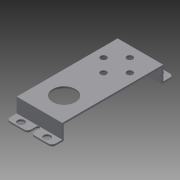
# Autodesk Inventor part: Quarter-Scale Servo Front Mount Bracket
Saved by Autodesk Inventor 2014 SP2 (Build 180246200, 246)
## iProperties
Created: 2014-09-14
Part Number: Quarter-Scale Servo Front Mount Bracket
Material: Generic
Document SubType Name: Modeling
Designer: Allison
Density: 1 g/cm^3
Appearance: Default
Author: Allison
Autodesk Inventor part; units mm, degrees
ref_plane "YZ Plane" through (0, 0, 0) normal (1, 0, 0) x (0, 1, 0)
ref_plane "XZ Plane" through (0, 0, 0) normal (0, 1, 0) x (-1, 0, 0)
ref_plane "XY Plane" through (0, 0, 0) normal (0, 0, 1) x (1, 0, 0)
sketch "Sketch1" plane through (0, 0, 0) normal (0, 1, 0) x (-1, 0, 0)
  line L0 (0.3746, 1.6788) -> (0.3747, -4.4196)
  line L1 (3.5497, -7.5946) -> (5.0483, -7.5946)
  arc A0 (7.6772, -6.364) -> (5.0483, -6.4323) centre (6.3183, -4.6863) ccw
  line L2 (7.6772, -7.5946) -> (20.7963, -7.5946)
  arc A1 (23.4251, -6.4323) -> (20.7962, -6.364) centre (22.1552, -4.6863) ccw
  line L3 (23.4252, -7.5946) -> (24.9238, -7.5946)
  line L4 (20.7963, 66.2432) -> (7.6772, 66.2432)
  arc A2 (5.0483, 65.0809) -> (7.6772, 65.0126) centre (6.3183, 63.3349) ccw
  line L5 (5.0483, 66.2432) -> (3.5496, 66.2432)
  line L6 (24.9237, 66.2432) -> (23.4252, 66.2432)
  arc A3 (20.7962, 65.0126) -> (23.4251, 65.0809) centre (22.1552, 63.3349) ccw
  circle A4 centre (14.2367, 45.0719) radius 6.9278
  arc A5 (1.9876, 15.9067) -> (5.1626, 12.7318) centre (5.1626, 15.9067) ccw
  line L7 (5.1626, 12.7318) -> (23.3109, 12.7318)
  arc A6 (23.3109, 12.7318) -> (26.4859, 15.9068) centre (23.3109, 15.9068) ccw
  line L8 (26.4859, 15.9068) -> (26.4859, 45.1707)
  arc A7 (26.4859, 45.1707) -> (1.9876, 45.1707) centre (14.2367, 45.0719) ccw
  line L9 (1.9876, 45.1707) -> (1.9876, 15.9067)
  arc A8 (27.813, 45.1759) -> (0.6604, 45.1759) centre (14.2367, 45.0719) ccw
  circle A9 centre (14.2367, 45.0719) radius 6.9278
  line L10 (0.3746, 66.2432) -> (13.2207, 66.2432)
  line L11 (13.2207, 66.2432) -> (13.2207, 60.019)
  line L12 (13.2207, 60.019) -> (0.3746, 60.019)
  line L13 (0.3746, 60.019) -> (0.3746, 66.2432)
  line L14 (0.3746, 60.019) -> (13.2207, 60.019)
  line L15 (13.2207, 60.019) -> (13.2207, 59.1663)
  line L16 (13.2207, 59.1663) -> (0.3746, 59.1663)
  line L17 (0.3746, 59.1663) -> (0.3746, 60.019)
  line L18 (14.2367, 45.0719) -> (14.2367, 66.2432)
  line L19 (28.0988, 66.2432) -> (15.2527, 66.2432)
  line L20 (15.2527, 66.2432) -> (15.2527, 60.019)
  line L21 (28.0988, 60.019) -> (28.0988, 66.2432)
  line L22 (28.0988, 60.019) -> (15.2527, 60.019)
  line L23 (15.2527, 60.019) -> (15.2527, 59.1663)
  line L24 (15.2527, 59.1663) -> (28.0988, 59.1663)
  line L25 (28.0988, 59.1663) -> (28.0988, 60.019)
  circle A10 centre (6.3183, 63.3349) radius 2.159
  circle A11 centre (22.1552, 63.3349) radius 2.159
  line L26 (0.3746, 66.2432) -> (0.3746, -7.5946)
  line L27 (0.3746, 29.3243) -> (28.0988, 29.3243)
  line L28 (20.7963, -7.5946) -> (7.6772, -7.5946)
  arc A12 (7.6772, -6.364) -> (5.0483, -6.4323) centre (6.3182, -4.6863) ccw
  line L29 (5.0483, -7.5946) -> (3.5497, -7.5946)
  line L30 (24.9238, -7.5946) -> (23.4252, -7.5946)
  arc A13 (23.4251, -6.4323) -> (20.7962, -6.364) centre (22.1551, -4.6863) ccw
  line L31 (0.3746, -7.5946) -> (13.2207, -7.5946)
  line L32 (13.2207, -7.5946) -> (13.2207, -1.3704)
  line L33 (13.2207, -1.3704) -> (0.3746, -1.3704)
  line L34 (0.3746, -1.3704) -> (0.3746, -7.5946)
  line L35 (0.3746, -1.3704) -> (13.2207, -1.3704)
  line L36 (13.2207, -1.3704) -> (13.2207, -0.5177)
  line L37 (13.2207, -0.5177) -> (0.3746, -0.5177)
  line L38 (0.3746, -0.5177) -> (0.3746, -1.3704)
  line L39 (28.0988, -1.3704) -> (28.0988, -7.5946)
  line L40 (28.0988, -7.5946) -> (15.2527, -7.5946)
  line L41 (15.2527, -7.5946) -> (15.2527, -1.3704)
  line L42 (28.0988, -1.3704) -> (15.2527, -1.3704)
  line L43 (15.2527, -0.5177) -> (28.0988, -0.5177)
  line L44 (15.2527, -1.3704) -> (15.2527, -0.5177)
  line L45 (28.0988, -0.5177) -> (28.0988, -1.3704)
  circle A14 centre (6.3182, -4.6863) radius 2.159
  circle A15 centre (22.1551, -4.6863) radius 2.159
  line L46 (28.0988, -7.5946) -> (15.2527, -7.5946)
  line L47 (15.2527, -7.5946) -> (15.2527, -1.3704)
  line L48 (15.2527, -1.3704) -> (28.0988, -1.3704)
  line L49 (28.0988, -1.3704) -> (28.0988, -7.5946)
  line L50 (13.2207, -7.5946) -> (0.3746, -7.5946)
  line L51 (0.3746, -7.5946) -> (0.3746, -1.3704)
  line L52 (0.3746, -1.3704) -> (13.2207, -1.3704)
  line L53 (13.2207, -1.3704) -> (13.2207, -7.5946)
  line L54 (28.0988, 66.2432) -> (15.2527, 66.2432)
  line L55 (15.2527, 66.2432) -> (15.2527, 60.019)
  line L56 (15.2527, 60.019) -> (28.0988, 60.019)
  line L57 (28.0988, 60.019) -> (28.0988, 66.2432)
  point P0 (0, 0)
  point P1 (0, 20.6785)
  point P2 (14.2367, -7.5946)
  constraints: 116 end point, 25 symmetric about line, 20 point on circle, 16 centre point, 11 parallel, 6 perpendicular, 5 horizontal, 4 coincident, 2 midpoint, 1 concentric, 4 other
extrude "Extrusion1" add sketch "Sketch1" along normal blind 1 contours L41 L42 L39 L40 L3 L2 | L4 L19 L6 L21 L22 L20 | L33 L32 L2 L31 L1 L26 L0 | L13 L10 L5 L4 L11 L12
sketch "Sketch2" plane through (0, 0, 0) normal (0, -1, 0) x (1, 0, 0)
  circle A0 centre (-22.1552, 63.3349) radius 2.159 projected
  line L0 (-28.0988, 66.2432) -> (-15.2527, 66.2432) projected
  line L1 (-28.0988, 60.019) -> (-28.0988, 66.2432) projected
  line L2 (-15.2527, 60.019) -> (-28.0988, 60.019) projected
  line L3 (-15.2527, 66.2432) -> (-15.2527, 60.019) projected
  circle A1 centre (-6.3183, 63.3349) radius 2.159 projected
  line L4 (-0.3746, 66.2432) -> (-0.3746, 60.019) projected
  line L5 (-13.2207, 66.2432) -> (-0.3746, 66.2432) projected
  line L6 (-13.2207, 60.019) -> (-13.2207, 66.2432) projected
  line L7 (-0.3746, 60.019) -> (-13.2207, 60.019) projected
  circle A2 centre (-22.1551, -4.6863) radius 2.159 projected
  line L8 (-15.2527, -1.3704) -> (-15.2527, -7.5946) projected
  line L9 (-28.0988, -1.3704) -> (-15.2527, -1.3704) projected
  line L10 (-28.0988, -7.5946) -> (-28.0988, -1.3704) projected
  line L11 (-15.2527, -7.5946) -> (-28.0988, -7.5946) projected
  line L12 (-28.0988, 60.019) -> (-0.3746, 60.019)
  line L13 (-0.3746, 60.019) -> (-0.3746, 59.13)
  line L14 (-0.3746, 59.13) -> (-28.0988, 59.13)
  line L15 (-28.0988, 59.13) -> (-28.0988, 60.019)
  line L16 (-28.0988, -1.3704) -> (-0.3746, -1.3704)
  line L17 (-0.3746, -1.3704) -> (-0.3746, -0.4814)
  line L18 (-0.3746, -0.4814) -> (-28.0988, -0.4814)
  line L19 (-28.0988, -0.4814) -> (-28.0988, -1.3704)
  point P0 (0, 0)
  dimension "d2" = 0.889
  dimension "d3" = 0.889
  constraints: 16 end point, 4 parallel, 2 horizontal, 2 perpendicular
  measures "d2" distance of L12.end L13.end
  measures "d3" distance of L17.end L16.end
extrude "Extrusion2" add sketch "Sketch2" against normal blind 8.8392 contours L2 L12 L7 L13 L14 L15 | L9 L19 L18 L17 L16
sketch "Sketch3" plane through (0, 8.8392, 0) normal (0, 1, 0) x (1, 0, 0)
  line L0 (-0.3746, 1.3704) -> (-28.0988, 1.3704)
  line L1 (-28.0988, 1.3704) -> (-28.0988, -60.019)
  line L2 (-28.0988, -60.019) -> (-0.3746, -60.019)
  line L3 (-0.3746, -60.019) -> (-0.3746, 1.3704)
  point P0 (0, 0)
  constraints: 8 end point, 2 parallel, 1 horizontal, 1 perpendicular
extrude "Extrusion3" add sketch "Sketch3" along normal blind 1
fillet "Fillet1" radius 2.032 8 edges at (-28.0988, 0.5, 66.2432) (-15.2527, 0.5, 66.2432) (-13.2207, 0.5, 66.2432) (-0.3746, 0.5, 66.2432) (-0.3746, 0.5, -7.5946) (-13.2207, 0.5, -7.5946) (-15.2527, 0.5, -7.5946) (-28.0988, 0.5, -7.5946)
fillet "Fillet2" radius 1.016 4 edges at (-13.2207, 0.5, -1.3704) (-15.2527, 0.5, -1.3704) (-15.2527, 0.5, 60.019) (-13.2207, 0.5, 60.019)
extrude "Extrusion4" cut sketch "Sketch1" along normal blind 127 contours A4
sketch "Sketch4" plane through (0, 9.8392, 0) normal (0, 1, 0) x (1, 0, 0)
  circle A0 centre (-14.2367, -45.0719) radius 6.9278 projected
  line L0 (-28.0988, 1.3704) -> (-28.0988, -60.019) projected
  circle A1 centre (-14.2367, -45.0719) radius 4.0005
  circle A2 centre (-14.2367, -13.0679) radius 4.0005
  line L1 (-14.2367, -13.0679) -> (-14.2367, -5.0669)
  circle A3 centre (-14.2367, -5.0669) radius 1.8542
  circle A4 centre (-22.2377, -13.0679) radius 1.8542
  circle A5 centre (-14.2367, -21.0689) radius 1.8542
  circle A6 centre (-6.2357, -13.0679) radius 1.8542
  point P0 (0, 0)
  dimension "d12" = 8.001
  dimension "d15" = 32.004
  dimension "d20" = 8.001
  dimension "d21" = 3.7084
  dimension "d24" = 360
  constraints: 6 centre point, 2 coincident, 2 end point, 1 parallel, 1 vertical, 11 other
  measures "d12" diameter of A1
  measures "d15" distance of A1.centre L1.start
  measures "d20" distance of L1.start L1.end
  measures "d21" diameter of A3
extrude "Extrusion5" cut sketch "Sketch4" against normal blind 127 contours A3 | A4 | A5 | A6
body "Solid1"
